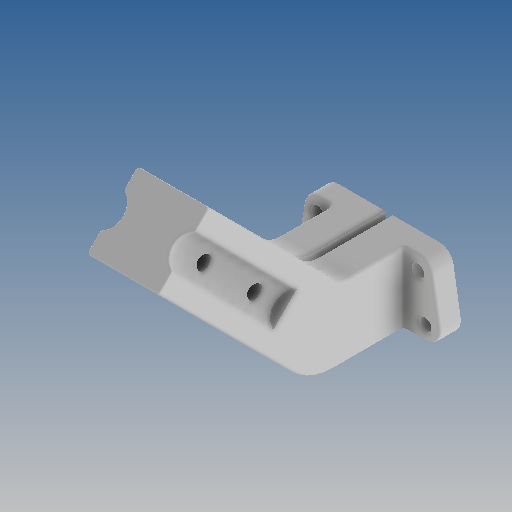
# Autodesk Inventor part: PWTR-0146
Saved by Autodesk Inventor 2021.1 (Build 251245000, 245)
## iProperties
Created: 2020-09-04
Part Number: PWTR-0146
Material: Generic
Document SubType Name: Modeling
Designer: alid
Density: 1 g/cm^3
Appearance: Default
Description: Lightweight Handle Base
Author: alid
Revision Number: A
Autodesk Inventor part; units mm, degrees
ref_plane "YZ Plane" through (0, 0, 0) normal (1, 0, 0) x (0, 1, 0)
ref_plane "XZ Plane" through (0, 0, 0) normal (0, 1, 0) x (-1, 0, 0)
ref_plane "XY Plane" through (0, 0, 0) normal (0, 0, 1) x (1, 0, 0)
sketch "Sketch2" plane through (0, 0, 0) normal (1, 0, 0) x (0, 1, 0)
  line L0 (0, 25) -> (0, -25)
  line L1 (0, 25) -> (-59.2893, 25)
  line L2 (-59.2893, 25) -> (-150.7107, 116.4214)
  line L3 (-150.7107, 116.4214) -> (-186.066, 81.066)
  line L4 (-186.066, 81.066) -> (-80, -25)
  line L5 (-80, -25) -> (0, -25)
  line L6 (-168.3883, 98.7437) -> (-111.8198, 42.1751) construction
  circle A0 centre (-111.8198, 42.1751) radius 5
  circle A1 centre (-147.1751, 77.5305) radius 5
  point P0 (0, 0)
  point P1 (0, 0)
  point P2 (0, 0)
  dimension "d3" = 50
  dimension "d4" = 80
  dimension "d5" = 135
  dimension "d6" = 150
  dimension "d7" = 50
  dimension "d8" = 80
  dimension "d34" = 10
  dimension "d41" = 50
  constraints: 14 end point, 3 coincident, 3 perpendicular, 2 centre point, 2 midpoint, 1 equal radius, 1 horizontal, 1 parallel, 1 point on line, 1 vertical
  measures "d3" distance of L0.start L0.end
  measures "d4" distance of L4.end L0.end
  measures "d5" angle of L4 L5
  measures "d6" distance of L3.end L4.end
  measures "d7" distance between parallel lines of L4 L2
  measures "d8" distance of L6.start L6.end
  measures "d34" diameter of A0
  measures "d41" distance of A1.centre A0.centre
extrude "Extrusion1" add sketch "Sketch2" along normal mid plane 50 contours L0 L5 L4 L3 L2 L1 | A0 | A1
sketch "Sketch3" plane through (0, 0, 0) normal (0, 1, 0) x (-1, 0, 0)
  line L0 (-40, -25) -> (40, -25)
  line L1 (35, 25) -> (-35, 25)
  line L2 (-49.8639, -13.356) -> (-44.8639, 16.644)
  line L3 (44.8639, 16.644) -> (49.8639, -13.356)
  circle A0 centre (-35, 15) radius 10
  circle A1 centre (-40, -15) radius 10
  circle A2 centre (35, 15) radius 10
  circle A3 centre (40, -15) radius 10
  line L4 (-35, 5) -> (35, 5)
  line L5 (-40, -5) -> (40, -5)
  line L6 (30.1361, -16.644) -> (25.1361, 13.356)
  line L7 (-25.1361, 13.356) -> (-30.1361, -16.644)
  point P0 (0, 0)
  point P1 (51.8046, -25)
  point P2 (0, 25)
  point P3 (0, -25)
  point P4 (0, -25)
  point P5 (-44.8639, 16.644)
  dimension "d11" = 70
  dimension "d12" = 50
  dimension "d13" = 25
  dimension "d14" = 80
  dimension "d15" = 20
  constraints: 16 end point, 16 tangent, 15 point on circle, 4 centre point, 3 coincident, 3 equal radius, 3 midpoint, 3 vertical alignment, 2 point on line, 1 equal length, 1 horizontal, 1 parallel
  measures "d11" distance of L1.start L1.end
  measures "d12" distance between parallel lines of L0 L1
  measures "d13" distance from line of L0 point (0, 0)
  measures "d14" distance of L0.start L0.end
  measures "d15" diameter of A0
extrude "Extrusion2" add sketch "Sketch3" against normal blind 15
hole "Hole1" at (-35, 0, 15) direction (0, -1, 0) diameter 9 end through all clearance for "Countersunk Flat Head Screw ISO 2009/7046" size "M8" standard "ISO"
pattern_sketch "Sketch Driven Pattern1" of "Hole1" from (-35, 0, 15) copies at (-40, 0, -15) at (40, 0, -15) at (35, 0, 15)
sketch "Sketch4" plane through (-25, -186.066, 81.066) normal (0, -0.7071068, 0.7071068) x (1, 0, 0)
  line L0 (0, 0) -> (50, 0) projected
  line L1 (50, 50) -> (50, 0) projected
  line L2 (50, 50) -> (0, 50) projected
  line L3 (0, 0) -> (0, 50) projected
  line L4 (25, 50) -> (25, 0) construction
  line L5 (25, 25) -> (-5, 25) construction
  circle A0 centre (-5, 25) radius 12.5
  point P0 (25, 74.2462)
  dimension "d25" = 30
  dimension "d26" = 25
  constraints: 4 end point, 3 midpoint, 1 centre point, 1 coincident, 1 horizontal
  measures "d25" distance of L5.start L5.end
  measures "d26" diameter of A0
extrude "Extrusion3" cut sketch "Sketch4" against normal blind 100 contours A0 L3 | L3 A0
mirror "Mirror1" about plane through (0, 0, 0) normal (1, 0, 0) of "Extrusion3"
fillet "Fillet1" radius 2 2 edges at (-25, -15, 0) (25, -15, 0)
fillet "Fillet2" radius 20 1 edges at (0, -59.2893, 25)
fillet "Fillet3" radius 40 1 edges at (0, -80, -25)
fillet "Fillet4" radius 2 30 edges at (-25, -58.6587, 26.5224) (-25, -34.0025, 25) (-25.5858, -15.5858, 25) (-31, -15, 25) (-41.4637, -15, 22.6302) (-47.3639, -15, 1.644) (-47.6302, -15, -21.4637) (-33.5, -15, -25) (-25.5858, -15.5858, -25) (-25, -40.2157, -25) (-25, -78.7388, -21.9552) (-25, -138.8909, 33.8909) (-25, -107.9289, 73.6396) (25, -58.6587, 26.5224) (25, -107.9289, 73.6396) (25.5858, -15.5858, 25) (31, -15, 25) (41.4637, -15, 22.6302) (47.3639, -15, 1.644) (47.6302, -15, -21.4637) (33.5, -15, -25) (25.5858, -15.5858, -25) (25, -40.2157, -25) (25, -78.7388, -21.9552) (25, -138.8909, 33.8909) (25, -34.0025, 25) (-25, -141.1332, 55.2867) (-25, -124.9314, 71.4886) (25, -141.1332, 55.2867) (25, -124.9314, 71.4886)
fillet "Fillet5" radius 1 16 edges at (0, -150.7107, 116.4214) (-24.4142, -151.1249, 116.0071) (-25, -155.767, 111.365) (-24.7221, -160.1284, 107.0036) (-24.7221, -176.6483, 90.4837) (-17.5, -168.3883, 98.7437) (-25, -181.0096, 86.1224) (-24.4142, -185.6518, 81.4802) (0, -186.066, 81.066) (24.4142, -185.6518, 81.4802) (25, -181.0096, 86.1224) (24.7221, -160.1284, 107.0036) (24.7221, -176.6483, 90.4837) (17.5, -168.3883, 98.7437) (25, -155.767, 111.365) (24.4142, -151.1249, 116.0071)
extrude "Extrusion4" cut sketch "Sketch2" along normal through all both and the other way through all contours A0 | A1
sketch "Sketch5" plane through (0, 0, 0) normal (0, 0, 1) x (1, 0, 0)
  line L0 (2.5, 0) -> (-2.5, 0)
  line L1 (-2.5, 0) -> (-2.5, -100)
  line L2 (-2.5, -100) -> (2.5, -100)
  line L3 (2.5, -100) -> (2.5, 0)
  point P0 (0, 0)
  point P1 (0, 0)
  dimension "d37" = 5
  dimension "d38" = 100
  constraints: 8 end point, 2 parallel, 1 coincident, 1 horizontal, 1 midpoint, 1 perpendicular
  measures "d37" distance of L2.end L1.end
  measures "d38" distance of L1.end L0.end
extrude "Extrusion5" cut sketch "Sketch5" along normal through all both and the other way through all
equation "\"d7\" = d3"
equation "\"d13\" = 0.5 * d12"
body "Solid1"
